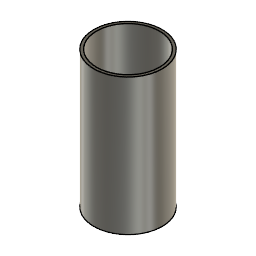
Rohr (Autodesk Fusion 360 design; units mm, degrees)
Autodesk Fusion 360 part; units mm, degrees
cylinder "Grundkörper Zylinder1" add diameter 25 height 50 placed x (1, 0, 0) y (0, 1, 0) z (0, 0, 1) at (0, 0, 0)
shell "Schale1" thickness 1 removed faces 2 at (-3.3879, -0.621, 50) at (-3.3879, -0.621, 0)
